Autodesk Fusion 360 part; units mm, degrees
note: some values were not read from the file. Chosen so that the rebuilt part matches the saved one: that a step has no effect.
(part 2 of 3)
sketch "Esquisse23" plane through (0, 78.1168, 0) normal (0, 1, 0) x (-1, 0, 0)
  arc A0 (-120.0939, -5.0643) -> (-115.0939, -10.0643) centre (-115.0939, -5.0643) ccw
  line L0 (-115.0939, -10.0643) -> (-5.0939, -10.0643)
  arc A1 (-5.0939, -10.0643) -> (-0.0939, -5.0643) centre (-5.0939, -5.0643) ccw
  line L1 (-0.0939, -5.0643) -> (-0.0939, 142.9357)
  arc A2 (-0.0939, 142.9357) -> (-5.0939, 147.9357) centre (-5.0939, 142.9357) ccw
  line L2 (-5.0939, 147.9357) -> (-115.0939, 147.9357)
  arc A3 (-115.0939, 147.9357) -> (-120.0939, 142.9357) centre (-115.0939, 142.9357) ccw
  line L3 (-120.0939, 142.9357) -> (-120.0939, -5.0643)
  line L4 (-52.5939, 55.5607) -> (-52.5939, 82.3107)
  line L5 (-52.5939, 82.3107) -> (-37.5939, 82.3107)
  line L6 (-37.5939, 82.3107) -> (-37.5939, 55.5607)
  line L7 (-37.5939, 55.5607) -> (-52.5939, 55.5607)
  circle A4 centre (-17.488, 58.9355) radius 2.625
  circle A5 centre (-17.4939, 78.9357) radius 2.6
  spline S0 degree 3 poles (-59.3641, 46.4248) (-58.9648, 44.9472) (-58.6266, 42.1699) (-58.7596, 41.7802) knots 0 0 0 0 1 1 1 1
  spline S1 degree 3 poles (-58.7596, 41.7802) (-58.8164, 41.6787) (-59.2704, 41.5542) (-59.7808, 41.5574) knots 0 0 0 0 1 1 1 1
  line L8 (-59.7808, 41.5574) -> (-60.6789, 41.5163)
  line L9 (-60.6789, 41.5163) -> (-60.7105, 42.3931)
  spline S2 degree 3 poles (-60.7105, 42.3931) (-60.7436, 43.9055) (-61.4034, 46.4895) (-62.2511, 48.405) knots 0 0 0 0 1 1 1 1
  spline S3 degree 3 poles (-62.2511, 48.405) (-64.5962, 53.7047) (-70.1315, 57.6435) (-75.845, 58.0167) knots 0 0 0 0 1 1 1 1
  spline S4 degree 3 poles (-75.845, 58.0167) (-77.6833, 58.1449) (-77.7447, 58.1686) (-77.7767, 58.8162) knots 0 0 0 0 1 1 1 1
  spline S5 degree 3 poles (-77.7767, 58.8162) (-77.8384, 60.1633) (-77.7414, 60.2317) (-75.8511, 60.101) knots 0 0 0 0 1 1 1 1
  spline S6 degree 3 poles (-75.8511, 60.101) (-74.9059, 60.0357) (-73.7057, 59.8541) (-73.2333, 59.7068) knots 0 0 0 0 1 1 1 1
  spline S7 degree 3 poles (-73.2333, 59.7068) (-72.7396, 59.569) (-71.9177, 59.3219) (-71.4121, 59.2147) knots 0 0 0 0 1 1 1 1
  spline S8 degree 3 poles (-71.4121, 59.2147) (-69.3523, 58.701) (-65.4571, 56.2252) (-63.7728, 54.3745) knots 0 0 0 0 1 1 1 1
  spline S9 degree 3 poles (-63.7728, 54.3745) (-63.367, 53.9177) (-62.7091, 53.0636) (-62.2988, 52.4816) knots 0 0 0 0 1 1 1 1
  spline S10 degree 3 poles (-62.2988, 52.4816) (-61.8886, 51.8996) (-61.4194, 51.2419) (-61.2732, 51.0266) knots 0 0 0 0 1 1 1 1
  spline S11 degree 3 poles (-61.2732, 51.0266) (-60.7168, 50.2293) (-59.7139, 47.848) (-59.3641, 46.4248) knots 0 0 0 0 1 1 1 1
  spline S12 degree 3 poles (-64.0578, 43.2279) (-63.857, 41.7388) (-63.895, 41.5947) (-64.3772, 41.5341) knots 0 0 0 0 1 1 1 1
  spline S13 degree 3 poles (-64.3772, 41.5341) (-65.2896, 41.4103) (-65.4382, 41.5736) (-65.639, 43.0627) knots 0 0 0 0 1 1 1 1
  spline S14 degree 3 poles (-65.639, 43.0627) (-65.9406, 45.0671) (-67.2358, 47.879) (-68.5238, 49.2943) knots 0 0 0 0 1 1 1 1
  spline S15 degree 3 poles (-68.5238, 49.2943) (-70.6445, 51.6136) (-73.2088, 52.9222) (-76.1859, 53.2082) knots 0 0 0 0 1 1 1 1
  spline S16 degree 3 poles (-76.1859, 53.2082) (-77.0153, 53.2993) (-77.698, 53.4044) (-77.7075, 53.4257) knots 0 0 0 0 1 1 1 1
  spline S17 degree 3 poles (-77.7075, 53.4257) (-77.8299, 53.7024) (-77.6934, 54.8318) (-77.5444, 54.8977) knots 0 0 0 0 1 1 1 1
  spline S18 degree 3 poles (-77.5444, 54.8977) (-76.991, 55.1426) (-74.5599, 54.7676) (-72.8996, 54.1789) knots 0 0 0 0 1 1 1 1
  spline S19 degree 3 poles (-72.8996, 54.1789) (-68.0508, 52.4814) (-64.782, 48.4304) (-64.0578, 43.2279) knots 0 0 0 0 1 1 1 1
  spline S20 degree 3 poles (-68.6528, 42.5689) (-68.581, 41.659) (-68.7398, 41.3851) (-69.3305, 41.4546) knots 0 0 0 0 1 1 1 1
  spline S21 degree 3 poles (-69.3305, 41.4546) (-69.6305, 41.5) (-69.7059, 41.6703) (-69.7944, 42.4455) knots 0 0 0 0 1 1 1 1
  spline S22 degree 3 poles (-69.7944, 42.4455) (-69.906, 43.6178) (-70.7724, 45.5759) (-71.5933, 46.5107) knots 0 0 0 0 1 1 1 1
  spline S23 degree 3 poles (-71.5933, 46.5107) (-72.6029, 47.6419) (-74.265, 48.6371) (-75.7296, 48.9562) knots 0 0 0 0 1 1 1 1
  spline S24 degree 3 poles (-75.7296, 48.9562) (-76.4619, 49.1157) (-77.1873, 49.2019) (-77.315, 49.1454) knots 0 0 0 0 1 1 1 1
  spline S25 degree 3 poles (-77.315, 49.1454) (-77.5917, 49.023) (-77.8013, 49.4392) (-77.7249, 49.9566) knots 0 0 0 0 1 1 1 1
  spline S26 degree 3 poles (-77.7249, 49.9566) (-77.677, 50.3087) (-77.5186, 50.3533) (-76.6774, 50.2929) knots 0 0 0 0 1 1 1 1
  spline S27 degree 3 poles (-76.6774, 50.2929) (-75.6283, 50.2226) (-73.453, 49.5055) (-72.5229, 48.899) knots 0 0 0 0 1 1 1 1
  spline S28 degree 3 poles (-72.5229, 48.899) (-70.7429, 47.7523) (-68.8079, 44.5873) (-68.6528, 42.5689) knots 0 0 0 0 1 1 1 1
  spline S29 degree 3 poles (-74.9422, 33.143) (-74.9747, 29.1328) (-75.0002, 25.0493) (-75.0041, 24.0804) knots 0 0 0 0 1 1 1 1
  spline S30 degree 3 poles (-75.0041, 24.0804) (-75.0199, 23.0808) (-75.059, 19.3731) (-75.0694, 15.8307) knots 0 0 0 0 1 1 1 1
  spline S31 degree 3 poles (-75.0694, 15.8307) (-75.1114, 10.2892) (-75.1862, 9.3653) (-75.5906, 9.1864) knots 0 0 0 0 1 1 1 1
  spline S32 degree 3 poles (-75.5906, 9.1864) (-76.2078, 8.9133) (-76.817, 9.2545) (-76.8891, 9.9352) knots 0 0 0 0 1 1 1 1
  spline S33 degree 3 poles (-76.8891, 9.9352) (-76.9383, 10.2189) (-76.9291, 11.521) (-76.9105, 12.8018) knots 0 0 0 0 1 1 1 1
  spline S34 degree 3 poles (-76.9105, 12.8018) (-76.838, 15.2263) (-76.7795, 22.2258) (-76.7274, 31.0805) knots 0 0 0 0 1 1 1 1
  spline S35 degree 3 poles (-76.7274, 31.0805) (-76.7275, 33.9565) (-76.6985, 37.227) (-76.6779, 38.3306) knots 0 0 0 0 1 1 1 1
  spline S36 degree 3 poles (-76.6779, 38.3306) (-76.6109, 41.7452) (-77.5591, 42.8527) (-80.4187, 42.7581) knots 0 0 0 0 1 1 1 1
  spline S37 degree 3 poles (-80.4187, 42.7581) (-81.2955, 42.7264) (-82.6307, 42.6955) (-83.401, 42.7109) knots 0 0 0 0 1 1 1 1
  spline S38 degree 3 poles (-83.401, 42.7109) (-87.5058, 42.727) (-93.9691, 42.6665) (-107.0636, 42.5222) knots 0 0 0 0 1 1 1 1
  spline S39 degree 3 poles (-107.0636, 42.5222) (-109.3583, 42.474) (-110.375, 42.1258) (-110.9864, 41.0918) knots 0 0 0 0 1 1 1 1
  spline S40 degree 3 poles (-110.9864, 41.0918) (-111.4296, 40.3103) (-111.4345, 40.2063) (-111.4267, 33.287) knots 0 0 0 0 1 1 1 1
  spline S41 degree 3 poles (-111.4267, 33.287) (-111.4378, 30.8388) (-111.4136, 28.2534) (-111.436, 27.5563) knots 0 0 0 0 1 1 1 1
  spline S42 degree 3 poles (-111.436, 27.5563) (-111.4418, 25.4413) (-111.443, 15.8965) (-111.4485, 5.1537) knots 0 0 0 0 1 1 1 1
  spline S43 degree 3 poles (-111.4485, 5.1537) (-111.441, -0.4423) (-111.4983, -5.2016) (-111.5388, -5.3977) knots 0 0 0 0 1 1 1 1
  spline S44 degree 3 poles (-111.5388, -5.3977) (-111.698, -5.9008) (-112.3553, -6.1408) (-112.7991, -5.8281) knots 0 0 0 0 1 1 1 1
  spline S45 degree 3 poles (-112.7991, -5.8281) (-113.231, -5.4848) (-113.2035, -6.0071) (-113.2071, 3.4338) knots 0 0 0 0 1 1 1 1
  spline S46 degree 3 poles (-113.2071, 3.4338) (-113.2025, 7.737) (-113.2023, 13.7182) (-113.2069, 16.7194) knots 0 0 0 0 1 1 1 1
  spline S47 degree 3 poles (-113.2069, 16.7194) (-113.1903, 19.73) (-113.1812, 23.9081) (-113.1967, 26.0137) knots 0 0 0 0 1 1 1 1
  spline S48 degree 3 poles (-113.1967, 26.0137) (-113.1815, 28.1074) (-113.1773, 32.1815) (-113.1892, 35.0267) knots 0 0 0 0 1 1 1 1
  spline S49 degree 3 poles (-113.1892, 35.0267) (-113.2201, 40.7905) (-112.989, 41.9363) (-111.5029, 43.1793) knots 0 0 0 0 1 1 1 1
  spline S50 degree 3 poles (-111.5029, 43.1793) (-110.3766, 44.0849) (-109.5445, 44.275) (-106.0115, 44.2858) knots 0 0 0 0 1 1 1 1
  spline S51 degree 3 poles (-106.0115, 44.2858) (-104.3857, 44.2926) (-102.436, 44.3155) (-101.6845, 44.3426) knots 0 0 0 0 1 1 1 1
  spline S52 degree 3 poles (-101.6845, 44.3426) (-100.9236, 44.3485) (-99.2031, 44.3717) (-97.8798, 44.3719) knots 0 0 0 0 1 1 1 1
  spline S53 degree 3 poles (-97.8798, 44.3719) (-96.5564, 44.3722) (-94.784, 44.3929) (-93.9498, 44.4058) knots 0 0 0 0 1 1 1 1
  spline S54 degree 3 poles (-93.9498, 44.4058) (-93.1156, 44.4186) (-91.7497, 44.4377) (-90.8966, 44.4079) knots 0 0 0 0 1 1 1 1
  spline S55 degree 3 poles (-90.8966, 44.4079) (-90.053, 44.3995) (-87.1132, 44.4278) (-84.36, 44.4754) knots 0 0 0 0 1 1 1 1
  spline S56 degree 3 poles (-84.36, 44.4754) (-77.5917, 44.5944) (-76.3092, 44.1693) (-75.3563, 41.6132) knots 0 0 0 0 1 1 1 1
  spline S57 degree 3 poles (-75.3563, 41.6132) (-74.9963, 40.6272) (-74.9232, 39.0816) (-74.9422, 33.143) knots 0 0 0 0 1 1 1 1
  spline S58 degree 3 poles (-107.0966, 36.7302) (-107.157, 35.889) (-107.6232, 35.5046) (-108.0408, 35.9306) knots 0 0 0 0 1 1 1 1
  spline S59 degree 3 poles (-108.0408, 35.9306) (-108.2107, 36.0845) (-108.5865, 36.0709) (-109.0003, 35.9133) knots 0 0 0 0 1 1 1 1
  line L10 (-109.0003, 35.9133) -> (-109.6695, 35.6426)
  line L11 (-109.6695, 35.6426) -> (-109.1251, 36.138)
  spline S60 degree 3 poles (-109.1251, 36.138) (-108.3938, 36.8434) (-108.3861, 37.2285) (-109.0807, 37.3029) knots 0 0 0 0 1 1 1 1
  spline S61 degree 3 poles (-109.0807, 37.3029) (-109.9526, 37.3752) (-109.1983, 37.6836) (-108.0616, 37.703) knots 0 0 0 0 1 1 1 1
  spline S62 degree 3 poles (-108.0616, 37.703) (-107.0194, 37.7061) (-107.0382, 37.7486) (-107.0966, 36.7302) knots 0 0 0 0 1 1 1 1
  spline S63 degree 3 poles (-107.2434, 33.6111) (-107.286, 33.5922) (-107.3564, 33.8665) (-107.3819, 34.2115) knots 0 0 0 0 1 1 1 1
  spline S64 degree 3 poles (-107.3819, 34.2115) (-107.416, 35.0363) (-107.4254, 35.0576) (-107.8085, 34.8881) knots 0 0 0 0 1 1 1 1
  spline S65 degree 3 poles (-107.8085, 34.8881) (-107.9575, 34.8222) (-108.1376, 34.5389) (-108.1711, 34.2695) knots 0 0 0 0 1 1 1 1
  spline S66 degree 3 poles (-108.1711, 34.2695) (-108.2426, 33.8561) (-108.2734, 33.868) (-108.3766, 34.3313) knots 0 0 0 0 1 1 1 1
  spline S67 degree 3 poles (-108.3766, 34.3313) (-108.4327, 34.6882) (-108.6427, 34.8753) (-109.0066, 34.8924) knots 0 0 0 0 1 1 1 1
  spline S68 degree 3 poles (-109.0066, 34.8924) (-109.7958, 34.9504) (-109.545, 35.1886) (-108.5925, 35.2793) knots 0 0 0 0 1 1 1 1
  spline S69 degree 3 poles (-108.5925, 35.2793) (-107.2429, 35.3929) (-107.0399, 35.2791) (-107.1122, 34.4072) knots 0 0 0 0 1 1 1 1
  spline S70 degree 3 poles (-107.1122, 34.4072) (-107.1317, 33.9914) (-107.2009, 33.6299) (-107.2434, 33.6111) knots 0 0 0 0 1 1 1 1
  spline S71 degree 3 poles (-107.1524, 32.8878) (-107.4504, 32.7559) (-109.6338, 32.8587) (-109.565, 32.9909) knots 0 0 0 0 1 1 1 1
  spline S72 degree 3 poles (-109.565, 32.9909) (-109.4701, 33.2366) (-107.2557, 33.3511) (-107.1521, 33.117) knots 0 0 0 0 1 1 1 1
  spline S73 degree 3 poles (-107.1521, 33.117) (-107.105, 33.0106) (-107.1099, 32.9066) (-107.1524, 32.8878) knots 0 0 0 0 1 1 1 1
  spline S74 degree 3 poles (-107.3093, 30.8841) (-107.5462, 30.4993) (-107.8135, 30.3556) (-108.2838, 30.3256) knots 0 0 0 0 1 1 1 1
  spline S75 degree 3 poles (-108.2838, 30.3256) (-109.0566, 30.289) (-109.5426, 30.8121) (-109.5341, 31.6557) knots 0 0 0 0 1 1 1 1
  spline S76 degree 3 poles (-109.5341, 31.6557) (-109.5285, 32.2181) (-109.4409, 32.3078) (-108.9399, 32.3259) knots 0 0 0 0 1 1 1 1
  spline S77 degree 3 poles (-108.9399, 32.3259) (-108.6161, 32.3419) (-108.0725, 32.3788) (-107.7487, 32.3949) knots 0 0 0 0 1 1 1 1
  spline S78 degree 3 poles (-107.7487, 32.3949) (-106.9972, 32.422) (-106.7928, 31.6726) (-107.3093, 30.8841) knots 0 0 0 0 1 1 1 1
  spline S79 degree 3 poles (-107.0664, 27.632) (-107.1494, 27.4171) (-107.3578, 27.1976) (-107.528, 27.1223) knots 0 0 0 0 1 1 1 1
  spline S80 degree 3 poles (-107.528, 27.1223) (-107.8354, 27.0117) (-107.833, 27.0637) (-107.6173, 27.4391) knots 0 0 0 0 1 1 1 1
  spline S81 degree 3 poles (-107.6173, 27.4391) (-107.2523, 28.1097) (-107.6577, 28.7956) (-108.3502, 28.6928) knots 0 0 0 0 1 1 1 1
  spline S82 degree 3 poles (-108.3502, 28.6928) (-109.1492, 28.5428) (-109.3649, 28.1674) (-108.9546, 27.5854) knots 0 0 0 0 1 1 1 1
  spline S83 degree 3 poles (-108.9546, 27.5854) (-108.7495, 27.2944) (-108.7474, 27.1172) (-108.9152, 27.0938) knots 0 0 0 0 1 1 1 1
  spline S84 degree 3 poles (-108.9152, 27.0938) (-109.7425, 27.0077) (-109.7469, 28.6856) (-108.8955, 29.0623) knots 0 0 0 0 1 1 1 1
  spline S85 degree 3 poles (-108.8955, 29.0623) (-108.0016, 29.4579) (-106.746, 28.4609) (-107.0664, 27.632) knots 0 0 0 0 1 1 1 1
  spline S86 degree 3 poles (-107.8998, 25.2017) (-108.3467, 25.0039) (-108.9378, 24.8441) (-109.219, 24.847) knots 0 0 0 0 1 1 1 1
  spline S87 degree 3 poles (-109.219, 24.847) (-109.6987, 24.8383) (-109.7081, 24.8596) (-109.2612, 25.0573) knots 0 0 0 0 1 1 1 1
  spline S88 degree 3 poles (-109.2612, 25.0573) (-108.7172, 25.3235) (-108.7489, 26.2003) (-109.2991, 26.4658) knots 0 0 0 0 1 1 1 1
  spline S89 degree 3 poles (-109.2991, 26.4658) (-110.0523, 26.8452) (-109.3552, 26.8228) (-108.3515, 26.4525) knots 0 0 0 0 1 1 1 1
  spline S90 degree 3 poles (-108.3515, 26.4525) (-107.0194, 25.973) (-106.89, 25.623) (-107.8998, 25.2017) knots 0 0 0 0 1 1 1 1
  spline S91 degree 3 poles (-107.4597, 22.5968) (-107.6631, 22.4813) (-107.9656, 22.4747) (-108.1568, 22.6191) knots 0 0 0 0 1 1 1 1
  spline S92 degree 3 poles (-108.1568, 22.6191) (-108.348, 22.7636) (-108.7545, 22.7619) (-109.0831, 22.6419) knots 0 0 0 0 1 1 1 1
  spline S93 degree 3 poles (-109.0831, 22.6419) (-109.4237, 22.4912) (-109.5583, 22.508) (-109.395, 22.6566) knots 0 0 0 0 1 1 1 1
  spline S94 degree 3 poles (-109.395, 22.6566) (-109.253, 22.7958) (-108.9359, 23.1143) (-108.685, 23.3526) knots 0 0 0 0 1 1 1 1
  line L12 (-108.685, 23.3526) -> (-108.2471, 23.8009)
  line L13 (-108.2471, 23.8009) -> (-108.9675, 23.9911)
  line L14 (-108.9675, 23.9911) -> (-109.6974, 24.2026)
  line L15 (-109.6974, 24.2026) -> (-109.0568, 24.3079)
  spline S95 degree 3 poles (-109.0568, 24.3079) (-108.7093, 24.3853) (-108.1231, 24.4411) (-107.7781, 24.4665) knots 0 0 0 0 1 1 1 1
  spline S96 degree 3 poles (-107.7781, 24.4665) (-107.1825, 24.501) (-107.1424, 24.4679) (-107.1271, 23.6856) knots 0 0 0 0 1 1 1 1
  spline S97 degree 3 poles (-107.1271, 23.6856) (-107.1066, 23.2366) (-107.2657, 22.7335) (-107.4597, 22.5968) knots 0 0 0 0 1 1 1 1
  spline S98 degree 3 poles (-107.1009, 20.9231) (-107.1515, 20.2898) (-108.185, 19.807) (-108.8817, 20.0587) knots 0 0 0 0 1 1 1 1
  spline S99 degree 3 poles (-108.8817, 20.0587) (-109.3824, 20.2698) (-109.7259, 21.1612) (-109.5218, 21.7352) knots 0 0 0 0 1 1 1 1
  spline S100 degree 3 poles (-109.5218, 21.7352) (-109.3794, 22.1036) (-107.3683, 22.1027) (-107.2082, 21.7409) knots 0 0 0 0 1 1 1 1
  spline S101 degree 3 poles (-107.2082, 21.7409) (-107.1329, 21.5706) (-107.098, 21.2043) (-107.1009, 20.9231) knots 0 0 0 0 1 1 1 1
  spline S102 degree 3 poles (-107.3413, 16.9226) (-107.41, 16.7904) (-107.7219, 16.8051) (-108.0195, 16.9025) knots 0 0 0 0 1 1 1 1
  spline S103 degree 3 poles (-108.0195, 16.9025) (-108.3265, 17.0211) (-108.7662, 16.9793) (-109.0453, 16.8049) knots 0 0 0 0 1 1 1 1
  spline S104 degree 3 poles (-109.0453, 16.8049) (-109.3457, 16.621) (-109.5229, 16.6189) (-109.5037, 16.8056) knots 0 0 0 0 1 1 1 1
  spline S105 degree 3 poles (-109.5037, 16.8056) (-109.4751, 16.971) (-109.2881, 17.181) (-109.0753, 17.2752) knots 0 0 0 0 1 1 1 1
  spline S106 degree 3 poles (-109.0753, 17.2752) (-108.8624, 17.3694) (-108.6304, 17.6502) (-108.5662, 17.9077) knots 0 0 0 0 1 1 1 1
  spline S107 degree 3 poles (-108.5662, 17.9077) (-108.4545, 18.288) (-108.504, 18.3424) (-108.9342, 18.2793) knots 0 0 0 0 1 1 1 1
  spline S108 degree 3 poles (-108.9342, 18.2793) (-109.4495, 18.1785) (-109.8106, 18.4768) (-109.4062, 18.6558) knots 0 0 0 0 1 1 1 1
  spline S109 degree 3 poles (-109.4062, 18.6558) (-109.2785, 18.7123) (-108.7042, 18.7374) (-108.1324, 18.7104) knots 0 0 0 0 1 1 1 1
  spline S110 degree 3 poles (-108.1324, 18.7104) (-107.114, 18.6521) (-107.1046, 18.6308) (-107.1507, 17.8723) knots 0 0 0 0 1 1 1 1
  spline S111 degree 3 poles (-107.1507, 17.8723) (-107.1703, 17.4564) (-107.2631, 17.0336) (-107.3413, 16.9226) knots 0 0 0 0 1 1 1 1
  spline S112 degree 3 poles (-107.1866, 14.675) (-107.2459, 14.5215) (-107.3286, 14.5358) (-107.4133, 14.7274) knots 0 0 0 0 1 1 1 1
  spline S113 degree 3 poles (-107.4133, 14.7274) (-107.4887, 14.8976) (-107.4953, 15.2001) (-107.4241, 15.3843) knots 0 0 0 0 1 1 1 1
  spline S114 degree 3 poles (-107.4241, 15.3843) (-107.2936, 15.7221) (-107.6285, 16.1338) (-107.9477, 15.9925) knots 0 0 0 0 1 1 1 1
  spline S115 degree 3 poles (-107.9477, 15.9925) (-108.0329, 15.9548) (-108.1114, 15.6147) (-108.1285, 15.2508) knots 0 0 0 0 1 1 1 1
  spline S116 degree 3 poles (-108.1285, 15.2508) (-108.115, 14.875) (-108.2005, 14.6081) (-108.2926, 14.6437) knots 0 0 0 0 1 1 1 1
  spline S117 degree 3 poles (-108.2926, 14.6437) (-108.3847, 14.6793) (-108.4457, 14.9323) (-108.4216, 15.2229) knots 0 0 0 0 1 1 1 1
  spline S118 degree 3 poles (-108.4216, 15.2229) (-108.3926, 15.6175) (-108.4892, 15.7783) (-108.8081, 15.8663) knots 0 0 0 0 1 1 1 1
  spline S119 degree 3 poles (-108.8081, 15.8663) (-109.1577, 15.9661) (-109.2359, 15.8552) (-109.2296, 15.3235) knots 0 0 0 0 1 1 1 1
  spline S120 degree 3 poles (-109.2296, 15.3235) (-109.2468, 14.9596) (-109.3253, 14.6194) (-109.4317, 14.5723) knots 0 0 0 0 1 1 1 1
  spline S121 degree 3 poles (-109.4317, 14.5723) (-109.5381, 14.5252) (-109.5967, 14.8301) (-109.5653, 15.2767) knots 0 0 0 0 1 1 1 1
  spline S122 degree 3 poles (-109.5653, 15.2767) (-109.5024, 16.1699) (-109.254, 16.3562) (-108.0157, 16.3187) knots 0 0 0 0 1 1 1 1
  spline S123 degree 3 poles (-108.0157, 16.3187) (-107.184, 16.2796) (-107.1344, 16.2252) (-107.1212, 15.6202) knots 0 0 0 0 1 1 1 1
  spline S124 degree 3 poles (-107.1212, 15.6202) (-107.1171, 15.2657) (-107.1367, 14.8498) (-107.1866, 14.675) knots 0 0 0 0 1 1 1 1
  spline S125 degree 3 poles (-108.3622, 12.5004) (-109.4902, 12.0013) (-110.1304, 12.1252) (-109.2292, 12.6767) knots 0 0 0 0 1 1 1 1
  spline S126 degree 3 poles (-109.2292, 12.6767) (-108.8531, 12.9195) (-108.8363, 13.0542) (-109.1827, 13.6644) knots 0 0 0 0 1 1 1 1
  line L16 (-109.1827, 13.6644) -> (-109.5762, 14.3811)
  line L17 (-109.5762, 14.3811) -> (-108.3575, 13.9278)
  spline S127 degree 3 poles (-108.3575, 13.9278) (-107.6821, 13.6667) (-107.1438, 13.3705) (-107.1605, 13.2358) knots 0 0 0 0 1 1 1 1
  spline S128 degree 3 poles (-107.1605, 13.2358) (-107.1867, 13.1224) (-107.7237, 12.783) (-108.3622, 12.5004) knots 0 0 0 0 1 1 1 1
  spline S129 degree 3 poles (-107.1618, 10.9955) (-107.2418, 9.7385) (-108.8635, 9.3772) (-109.3533, 10.4839) knots 0 0 0 0 1 1 1 1
  spline S130 degree 3 poles (-109.3533, 10.4839) (-109.8242, 11.5481) (-109.6347, 11.8101) (-108.3396, 11.8742) knots 0 0 0 0 1 1 1 1
  spline S131 degree 3 poles (-108.3396, 11.8742) (-107.7133, 11.8968) (-107.1722, 11.8817) (-107.1533, 11.8392) knots 0 0 0 0 1 1 1 1
  spline S132 degree 3 poles (-107.1533, 11.8392) (-107.1345, 11.7966) (-107.1422, 11.4114) (-107.1618, 10.9955) knots 0 0 0 0 1 1 1 1
  spline S133 degree 3 poles (-107.2947, 7.7299) (-107.3561, 7.7536) (-107.4147, 8.0585) (-107.4401, 8.4036) knots 0 0 0 0 1 1 1 1
  spline S134 degree 3 poles (-107.4401, 8.4036) (-107.4833, 9.4789) (-108.1214, 9.4256) (-108.1421, 8.322) knots 0 0 0 0 1 1 1 1
  spline S135 degree 3 poles (-108.1421, 8.322) (-108.1498, 7.9369) (-108.2541, 7.7125) (-108.3626, 7.8427) knots 0 0 0 0 1 1 1 1
  spline S136 degree 3 poles (-108.3626, 7.8427) (-108.4711, 7.9728) (-108.5604, 8.2896) (-108.5269, 8.559) knots 0 0 0 0 1 1 1 1
  spline S137 degree 3 poles (-108.5269, 8.559) (-108.4979, 8.9536) (-108.5757, 9.0719) (-108.8569, 9.0747) knots 0 0 0 0 1 1 1 1
  spline S138 degree 3 poles (-108.8569, 9.0747) (-109.0767, 9.0538) (-109.2355, 8.7799) (-109.2669, 8.3333) knots 0 0 0 0 1 1 1 1
  spline S139 degree 3 poles (-109.2669, 8.3333) (-109.3581, 7.504) (-109.6316, 7.892) (-109.5711, 8.7332) knots 0 0 0 0 1 1 1 1
  spline S140 degree 3 poles (-109.5711, 8.7332) (-109.5352, 9.0545) (-109.5111, 9.3451) (-109.5086, 9.3971) knots 0 0 0 0 1 1 1 1
  spline S141 degree 3 poles (-109.5086, 9.3971) (-109.4967, 9.4278) (-108.9626, 9.486) (-108.3056, 9.4968) knots 0 0 0 0 1 1 1 1
  line L18 (-108.3056, 9.4968) -> (-107.1382, 9.5044)
  line L19 (-107.1382, 9.5044) -> (-107.161, 8.578)
  spline S142 degree 3 poles (-107.161, 8.578) (-107.1736, 8.0889) (-107.2333, 7.7061) (-107.2947, 7.7299) knots 0 0 0 0 1 1 1 1
  spline S143 degree 3 poles (-107.1486, 5.962) (-107.3078, 5.4589) (-108.029, 5.1907) (-108.2079, 5.5951) knots 0 0 0 0 1 1 1 1
  spline S144 degree 3 poles (-108.2079, 5.5951) (-108.3209, 5.8505) (-108.4888, 5.8271) (-108.9312, 5.5041) knots 0 0 0 0 1 1 1 1
  spline S145 degree 3 poles (-108.9312, 5.5041) (-109.2979, 5.24) (-109.5414, 5.1577) (-109.6074, 5.3066) knots 0 0 0 0 1 1 1 1
  spline S146 degree 3 poles (-109.6074, 5.3066) (-109.6639, 5.4343) (-109.4769, 5.6444) (-109.2002, 5.7668) knots 0 0 0 0 1 1 1 1
  spline S147 degree 3 poles (-109.2002, 5.7668) (-108.9235, 5.8892) (-108.6395, 6.1676) (-108.5871, 6.3944) knots 0 0 0 0 1 1 1 1
  spline S148 degree 3 poles (-108.5871, 6.3944) (-108.4873, 6.744) (-108.5769, 6.8316) (-109.0235, 6.863) knots 0 0 0 0 1 1 1 1
  spline S149 degree 3 poles (-109.0235, 6.863) (-110.0207, 6.9308) (-109.5168, 7.2301) (-108.3376, 7.2684) knots 0 0 0 0 1 1 1 1
  spline S150 degree 3 poles (-108.3376, 7.2684) (-107.1583, 7.3067) (-106.8918, 6.9919) (-107.1486, 5.962) knots 0 0 0 0 1 1 1 1
  spline S151 degree 3 poles (-107.7762, 37.3457) (-108.0975, 37.3817) (-108.2804, 36.8172) (-108.0732, 36.3489) knots 0 0 0 0 1 1 1 1
  spline S152 degree 3 poles (-108.0732, 36.3489) (-107.9037, 35.9658) (-107.3573, 36.284) (-107.3872, 36.7543) knots 0 0 0 0 1 1 1 1
  spline S153 degree 3 poles (-107.3872, 36.7543) (-107.4147, 37.2766) (-107.4242, 37.2979) (-107.7762, 37.3457) knots 0 0 0 0 1 1 1 1
  spline S154 degree 3 poles (-108.0495, 31.9818) (-109.0209, 31.9337) (-109.3332, 31.7192) (-109.1448, 31.2935) knots 0 0 0 0 1 1 1 1
  spline S155 degree 3 poles (-109.1448, 31.2935) (-108.7586, 30.4209) (-107.5225, 30.5607) (-107.4477, 31.4846) knots 0 0 0 0 1 1 1 1
  spline S156 degree 3 poles (-107.4477, 31.4846) (-107.4163, 31.9311) (-107.5059, 32.0187) (-108.0495, 31.9818) knots 0 0 0 0 1 1 1 1
  spline S157 degree 3 poles (-108.0403, 25.9794) (-108.227, 25.9986) (-108.4067, 25.9445) (-108.4423, 25.8524) knots 0 0 0 0 1 1 1 1
  spline S158 degree 3 poles (-108.4423, 25.8524) (-108.549, 25.5761) (-108.1782, 25.4857) (-107.9273, 25.724) knots 0 0 0 0 1 1 1 1
  spline S159 degree 3 poles (-107.9273, 25.724) (-107.7309, 25.9127) (-107.7497, 25.9553) (-108.0403, 25.9794) knots 0 0 0 0 1 1 1 1
  spline S160 degree 3 poles (-107.7739, 24.112) (-108.0953, 24.148) (-108.2781, 23.5835) (-108.0709, 23.1153) knots 0 0 0 0 1 1 1 1
  spline S161 degree 3 poles (-108.0709, 23.1153) (-107.9297, 22.796) (-107.6648, 22.8878) (-107.475, 23.379) knots 0 0 0 0 1 1 1 1
  spline S162 degree 3 poles (-107.475, 23.379) (-107.297, 23.8395) (-107.3912, 24.0523) (-107.7739, 24.112) knots 0 0 0 0 1 1 1 1
  spline S163 degree 3 poles (-108.1726, 21.6196) (-109.0871, 21.673) (-109.4161, 21.3238) (-109.0058, 20.7418) knots 0 0 0 0 1 1 1 1
  spline S164 degree 3 poles (-109.0058, 20.7418) (-108.6357, 20.193) (-107.7422, 20.3593) (-107.5237, 21.0159) knots 0 0 0 0 1 1 1 1
  spline S165 degree 3 poles (-107.5237, 21.0159) (-107.3527, 21.5497) (-107.3834, 21.5616) (-108.1726, 21.6196) knots 0 0 0 0 1 1 1 1
  spline S166 degree 3 poles (-107.8376, 18.3319) (-108.1782, 18.1812) (-108.1702, 17.243) (-107.8325, 17.1125) knots 0 0 0 0 1 1 1 1
  spline S167 degree 3 poles (-107.8325, 17.1125) (-107.6176, 17.0294) (-107.323, 17.9742) (-107.4643, 18.2935) knots 0 0 0 0 1 1 1 1
  spline S168 degree 3 poles (-107.4643, 18.2935) (-107.502, 18.3786) (-107.6673, 18.4072) (-107.8376, 18.3319) knots 0 0 0 0 1 1 1 1
  spline S169 degree 3 poles (-108.1078, 13.4784) (-108.2944, 13.4976) (-108.4741, 13.4435) (-108.5097, 13.3514) knots 0 0 0 0 1 1 1 1
  spline S170 degree 3 poles (-108.5097, 13.3514) (-108.6165, 13.0751) (-108.2456, 12.9847) (-107.9947, 13.223) knots 0 0 0 0 1 1 1 1
  spline S171 degree 3 poles (-107.9947, 13.223) (-107.7983, 13.4117) (-107.8171, 13.4543) (-108.1078, 13.4784) knots 0 0 0 0 1 1 1 1
  spline S172 degree 3 poles (-108.3285, 11.4464) (-109.4369, 11.3631) (-109.4795, 11.3443) (-109.2158, 10.7484) knots 0 0 0 0 1 1 1 1
  spline S173 degree 3 poles (-109.2158, 10.7484) (-108.9897, 10.2376) (-108.5362, 10.1328) (-107.8125, 10.4531) knots 0 0 0 0 1 1 1 1
  spline S174 degree 3 poles (-107.8125, 10.4531) (-107.5146, 10.5849) (-107.3435, 11.1187) (-107.4942, 11.4593) knots 0 0 0 0 1 1 1 1
  spline S175 degree 3 poles (-107.4942, 11.4593) (-107.5037, 11.4805) (-107.8794, 11.467) (-108.3285, 11.4464) knots 0 0 0 0 1 1 1 1
  spline S176 degree 3 poles (-107.8774, 6.8612) (-108.2818, 6.6822) (-108.2899, 6.0678) (-107.8956, 5.8096) knots 0 0 0 0 1 1 1 1
  spline S177 degree 3 poles (-107.8956, 5.8096) (-107.7045, 5.6651) (-107.5956, 5.7642) (-107.5052, 6.1351) knots 0 0 0 0 1 1 1 1
  spline S178 degree 3 poles (-107.5052, 6.1351) (-107.3694, 6.806) (-107.473, 7.0401) (-107.8774, 6.8612) knots 0 0 0 0 1 1 1 1
  line L20 (-172.7478, 135.2795) -> (-285.7692, 135.2795)
  line L21 (-285.7692, 135.2795) -> (-285.7692, -50.5423)
  line L22 (-285.7692, -50.5423) -> (-172.7478, -50.5423)
  line L23 (-172.7478, -50.5423) -> (-172.7478, 135.2795)
  constraint horizontal L20
  constraint vertical L21
  constraint horizontal L22
  constraint vertical L23
sketch "Esquisse24" plane through (0, 78.1168, 0) normal (0, 1, 0) x (-1, 0, 0)
  arc A0 (-120.0939, -5.0643) -> (-115.0939, -10.0643) centre (-115.0939, -5.0643) ccw
  line L0 (-115.0939, -10.0643) -> (-5.0939, -10.0643)
  arc A1 (-5.0939, -10.0643) -> (-0.0939, -5.0643) centre (-5.0939, -5.0643) ccw
  line L1 (-0.0939, -5.0643) -> (-0.0939, 142.9357)
  arc A2 (-0.0939, 142.9357) -> (-5.0939, 147.9357) centre (-5.0939, 142.9357) ccw
  line L2 (-5.0939, 147.9357) -> (-115.0939, 147.9357)
  arc A3 (-115.0939, 147.9357) -> (-120.0939, 142.9357) centre (-115.0939, 142.9357) ccw
  line L3 (-120.0939, 142.9357) -> (-120.0939, -5.0643)
  line L4 (-52.5939, 55.5607) -> (-52.5939, 82.3107)
  line L5 (-52.5939, 82.3107) -> (-37.5939, 82.3107)
  line L6 (-37.5939, 82.3107) -> (-37.5939, 55.5607)
  line L7 (-37.5939, 55.5607) -> (-52.5939, 55.5607)
  circle A4 centre (-17.488, 58.9355) radius 2.625
  circle A5 centre (-17.4939, 78.9357) radius 2.6
  spline S0 degree 3 poles (-61.7818, 46.0045) (-61.433, 44.7265) (-61.1344, 42.3234) (-61.2487, 41.9858) knots 0 0 0 0 1 1 1 1
  spline S1 degree 3 poles (-61.2487, 41.9858) (-61.2977, 41.8978) (-61.6903, 41.7891) (-62.1321, 41.7907) knots 0 0 0 0 1 1 1 1
  line L8 (-62.1321, 41.7907) -> (-62.9094, 41.7533)
  line L9 (-62.9094, 41.7533) -> (-62.9386, 42.5121)
  spline S2 degree 3 poles (-62.9386, 42.5121) (-62.9704, 43.8211) (-63.547, 46.0563) (-64.2847, 47.7124) knots 0 0 0 0 1 1 1 1
  spline S3 degree 3 poles (-64.2847, 47.7124) (-66.3257, 52.2945) (-71.125, 55.692) (-76.071, 56.0029) knots 0 0 0 0 1 1 1 1
  spline S4 degree 3 poles (-76.071, 56.0029) (-77.6624, 56.11) (-77.7156, 56.1304) (-77.7447, 56.6908) knots 0 0 0 0 1 1 1 1
  spline S5 degree 3 poles (-77.7447, 56.6908) (-77.8009, 57.8566) (-77.7171, 57.916) (-76.0807, 57.8069) knots 0 0 0 0 1 1 1 1
  spline S6 degree 3 poles (-76.0807, 57.8069) (-75.2625, 57.7524) (-74.2233, 57.5978) (-73.8141, 57.4713) knots 0 0 0 0 1 1 1 1
  spline S7 degree 3 poles (-73.8141, 57.4713) (-73.3866, 57.353) (-72.6746, 57.1409) (-72.2368, 57.0492) knots 0 0 0 0 1 1 1 1
  spline S8 degree 3 poles (-72.2368, 57.0492) (-70.4528, 56.6089) (-67.0762, 54.4742) (-65.6144, 52.876) knots 0 0 0 0 1 1 1 1
  spline S9 degree 3 poles (-65.6144, 52.876) (-65.2623, 52.4815) (-64.691, 51.7436) (-64.3347, 51.2407) knots 0 0 0 0 1 1 1 1
  spline S10 degree 3 poles (-64.3347, 51.2407) (-63.9784, 50.7378) (-63.5709, 50.1695) (-63.4439, 49.9835) knots 0 0 0 0 1 1 1 1
  spline S11 degree 3 poles (-63.4439, 49.9835) (-62.9606, 49.2946) (-62.0876, 47.2356) (-61.7818, 46.0045) knots 0 0 0 0 1 1 1 1
  spline S12 degree 3 poles (-65.8375, 43.2276) (-65.6606, 41.9392) (-65.6932, 41.8144) (-66.1104, 41.7608) knots 0 0 0 0 1 1 1 1
  spline S13 degree 3 poles (-66.1104, 41.7608) (-66.8998, 41.6518) (-67.0288, 41.7928) (-67.2058, 43.0813) knots 0 0 0 0 1 1 1 1
  spline S14 degree 3 poles (-67.2058, 43.0813) (-67.4711, 44.8155) (-68.5981, 47.2466) (-69.7159, 48.4688) knots 0 0 0 0 1 1 1 1
  spline S15 degree 3 poles (-69.7159, 48.4688) (-71.5563, 50.4718) (-73.7786, 51.599) (-76.356, 51.8403) knots 0 0 0 0 1 1 1 1
  spline S16 degree 3 poles (-76.356, 51.8403) (-77.074, 51.9174) (-77.6652, 52.0069) (-77.6734, 52.0253) knots 0 0 0 0 1 1 1 1
  spline S17 degree 3 poles (-77.6734, 52.0253) (-77.7799, 52.2645) (-77.6642, 53.2423) (-77.5354, 53.2997) knots 0 0 0 0 1 1 1 1
  spline S18 degree 3 poles (-77.5354, 53.2997) (-77.0569, 53.5128) (-74.9519, 53.1934) (-73.5136, 52.6874) knots 0 0 0 0 1 1 1 1
  spline S19 degree 3 poles (-73.5136, 52.6874) (-69.3132, 51.2284) (-66.4753, 47.729) (-65.8375, 43.2276) knots 0 0 0 0 1 1 1 1
  spline S20 degree 3 poles (-69.8133, 42.6475) (-69.7493, 41.8601) (-69.8861, 41.6227) (-70.3975, 41.6816) knots 0 0 0 0 1 1 1 1
  spline S21 degree 3 poles (-70.3975, 41.6816) (-70.6573, 41.7203) (-70.7229, 41.8675) (-70.8012, 42.5383) knots 0 0 0 0 1 1 1 1
  spline S22 degree 3 poles (-70.8012, 42.5383) (-70.9002, 43.5527) (-71.6543, 45.2457) (-72.3668, 46.053) knots 0 0 0 0 1 1 1 1
  spline S23 degree 3 poles (-72.3668, 46.053) (-73.243, 47.03) (-74.6837, 47.8879) (-75.952, 48.1609) knots 0 0 0 0 1 1 1 1
  spline S24 degree 3 poles (-75.952, 48.1609) (-76.5862, 48.2974) (-77.2142, 48.3705) (-77.3246, 48.3214) knots 0 0 0 0 1 1 1 1
  spline S25 degree 3 poles (-77.3246, 48.3214) (-77.5639, 48.2148) (-77.7462, 48.5746) (-77.6811, 49.0226) knots 0 0 0 0 1 1 1 1
  spline S26 degree 3 poles (-77.6811, 49.0226) (-77.6405, 49.3274) (-77.5035, 49.3664) (-76.7752, 49.3159) knots 0 0 0 0 1 1 1 1
  spline S27 degree 3 poles (-76.7752, 49.3159) (-75.867, 49.2573) (-73.9827, 48.6412) (-73.1764, 48.1182) knots 0 0 0 0 1 1 1 1
  spline S28 degree 3 poles (-73.1764, 48.1182) (-71.6333, 47.1295) (-69.9518, 44.3942) (-69.8133, 42.6475) knots 0 0 0 0 1 1 1 1
  spline S29 degree 3 poles (-75.2371, 34.4757) (-75.2567, 31.0047) (-75.2701, 27.4702) (-75.2715, 26.6316) knots 0 0 0 0 1 1 1 1
  spline S30 degree 3 poles (-75.2715, 26.6316) (-75.283, 25.7664) (-75.309, 22.5571) (-75.3106, 19.4911) knots 0 0 0 0 1 1 1 1
  spline S31 degree 3 poles (-75.3106, 19.4911) (-75.3352, 14.6946) (-75.398, 13.8948) (-75.7476, 13.7391) knots 0 0 0 0 1 1 1 1
  spline S32 degree 3 poles (-75.7476, 13.7391) (-76.2812, 13.5014) (-76.8092, 13.7955) (-76.8731, 14.3845) knots 0 0 0 0 1 1 1 1
  spline S33 degree 3 poles (-76.8731, 14.3845) (-76.9163, 14.6299) (-76.9111, 15.7569) (-76.8977, 16.8655) knots 0 0 0 0 1 1 1 1
  spline S34 degree 3 poles (-76.8977, 16.8655) (-76.8401, 18.9642) (-76.8042, 25.0227) (-76.7778, 32.6868) knots 0 0 0 0 1 1 1 1
  spline S35 degree 3 poles (-76.7778, 32.6868) (-76.784, 35.176) (-76.7659, 38.0069) (-76.7503, 38.9621) knots 0 0 0 0 1 1 1 1
  spline S36 degree 3 poles (-76.7503, 38.9621) (-76.6996, 41.9177) (-77.5226, 42.8743) (-79.9975, 42.7863) knots 0 0 0 0 1 1 1 1
  spline S37 degree 3 poles (-79.9975, 42.7863) (-80.7563, 42.7571) (-81.9119, 42.7275) (-82.5787, 42.7392) knots 0 0 0 0 1 1 1 1
  spline S38 degree 3 poles (-82.5787, 42.7392) (-86.1316, 42.7444) (-91.7257, 42.6784) (-103.0591, 42.5259) knots 0 0 0 0 1 1 1 1
  spline S39 degree 3 poles (-103.0591, 42.5259) (-105.0452, 42.4792) (-105.9244, 42.1758) (-106.4514, 41.2794) knots 0 0 0 0 1 1 1 1
  spline S40 degree 3 poles (-106.4514, 41.2794) (-106.8333, 40.6021) (-106.8374, 40.5121) (-106.816, 34.5232) knots 0 0 0 0 1 1 1 1
  spline S41 degree 3 poles (-106.816, 34.5232) (-106.8204, 32.4042) (-106.794, 30.1665) (-106.8119, 29.5631) knots 0 0 0 0 1 1 1 1
  spline S42 degree 3 poles (-106.8119, 29.5631) (-106.8124, 27.7325) (-106.7933, 19.4711) (-106.7754, 10.1727) knots 0 0 0 0 1 1 1 1
  spline S43 degree 3 poles (-106.7754, 10.1727) (-106.7571, 5.3293) (-106.7966, 1.2098) (-106.8312, 1.04) knots 0 0 0 0 1 1 1 1
  spline S44 degree 3 poles (-106.8312, 1.04) (-106.9679, 0.6042) (-107.5363, 0.3951) (-107.9211, 0.6648) knots 0 0 0 0 1 1 1 1
  spline S45 degree 3 poles (-107.9211, 0.6648) (-108.2957, 0.9611) (-108.2707, 0.509) (-108.2939, 8.6804) knots 0 0 0 0 1 1 1 1
  spline S46 degree 3 poles (-108.2939, 8.6804) (-108.299, 12.4051) (-108.3115, 17.582) (-108.3218, 20.1796) knots 0 0 0 0 1 1 1 1
  spline S47 degree 3 poles (-108.3218, 20.1796) (-108.3138, 22.7854) (-108.3147, 26.4017) (-108.3326, 28.2242) knots 0 0 0 0 1 1 1 1
  spline S48 degree 3 poles (-108.3326, 28.2242) (-108.3239, 30.0364) (-108.3288, 33.5626) (-108.3452, 36.0253) knots 0 0 0 0 1 1 1 1
  spline S49 degree 3 poles (-108.3452, 36.0253) (-108.3841, 41.014) (-108.1865, 42.0062) (-106.9029, 43.0852) knots 0 0 0 0 1 1 1 1
  spline S50 degree 3 poles (-106.9029, 43.0852) (-105.9299, 43.8714) (-105.2101, 44.0377) (-102.1522, 44.0545) knots 0 0 0 0 1 1 1 1
  spline S51 degree 3 poles (-102.1522, 44.0545) (-100.745, 44.0639) (-99.0576, 44.0878) (-98.4072, 44.1129) knots 0 0 0 0 1 1 1 1
  spline S52 degree 3 poles (-98.4072, 44.1129) (-97.7486, 44.1195) (-96.2595, 44.1433) (-95.1141, 44.1463) knots 0 0 0 0 1 1 1 1
  spline S53 degree 3 poles (-95.1141, 44.1463) (-93.9687, 44.1493) (-92.4346, 44.171) (-91.7126, 44.1839) knots 0 0 0 0 1 1 1 1
  spline S54 degree 3 poles (-91.7126, 44.1839) (-90.9906, 44.1967) (-89.8084, 44.2161) (-89.07, 44.1922) knots 0 0 0 0 1 1 1 1
  spline S55 degree 3 poles (-89.07, 44.1922) (-88.3398, 44.1867) (-85.7953, 44.2174) (-83.4125, 44.2644) knots 0 0 0 0 1 1 1 1
  spline S56 degree 3 poles (-83.4125, 44.2644) (-77.5545, 44.3817) (-76.4436, 44.0165) (-75.6134, 41.8061) knots 0 0 0 0 1 1 1 1
  spline S57 degree 3 poles (-75.6134, 41.8061) (-75.2997, 40.9535) (-75.2332, 39.6158) (-75.2371, 34.4757) knots 0 0 0 0 1 1 1 1
  spline S58 degree 3 poles (-103.0754, 37.5126) (-103.126, 36.7844) (-103.5286, 36.4506) (-103.891, 36.8185) knots 0 0 0 0 1 1 1 1
  spline S59 degree 3 poles (-103.891, 36.8185) (-104.0383, 36.9513) (-104.3636, 36.9388) (-104.7214, 36.8015) knots 0 0 0 0 1 1 1 1
  line L10 (-104.7214, 36.8015) -> (-105.3, 36.5658)
  line L11 (-105.3, 36.5658) -> (-104.83, 36.9957)
  spline S60 degree 3 poles (-104.83, 36.9957) (-104.1984, 37.6078) (-104.1926, 37.9412) (-104.794, 38.0041) knots 0 0 0 0 1 1 1 1
  spline S61 degree 3 poles (-104.794, 38.0041) (-105.5488, 38.0648) (-104.8965, 38.3333) (-103.9127, 38.3525) knots 0 0 0 0 1 1 1 1
  spline S62 degree 3 poles (-103.9127, 38.3525) (-103.0107, 38.3574) (-103.0271, 38.3942) (-103.0754, 37.5126) knots 0 0 0 0 1 1 1 1
  spline S63 degree 3 poles (-103.1959, 34.8126) (-103.2327, 34.7962) (-103.2943, 35.0334) (-103.317, 35.332) knots 0 0 0 0 1 1 1 1
  spline S64 degree 3 poles (-103.317, 35.332) (-103.3483, 36.0458) (-103.3565, 36.0642) (-103.6877, 35.9167) knots 0 0 0 0 1 1 1 1
  spline S65 degree 3 poles (-103.6877, 35.9167) (-103.8165, 35.8593) (-103.9718, 35.6137) (-104.0002, 35.3805) knots 0 0 0 0 1 1 1 1
  spline S66 degree 3 poles (-104.0002, 35.3805) (-104.0613, 35.0225) (-104.0879, 35.0327) (-104.1782, 35.4335) knots 0 0 0 0 1 1 1 1
  spline S67 degree 3 poles (-104.1782, 35.4335) (-104.2276, 35.7424) (-104.4097, 35.9038) (-104.7247, 35.9178) knots 0 0 0 0 1 1 1 1
  spline S68 degree 3 poles (-104.7247, 35.9178) (-105.4079, 35.9664) (-105.1913, 36.1731) (-104.3671, 36.2536) knots 0 0 0 0 1 1 1 1
  spline S69 degree 3 poles (-104.3671, 36.2536) (-103.1992, 36.3548) (-103.0233, 36.2567) (-103.084, 35.5019) knots 0 0 0 0 1 1 1 1
  spline S70 degree 3 poles (-103.084, 35.5019) (-103.1001, 35.1419) (-103.1591, 34.8289) (-103.1959, 34.8126) knots 0 0 0 0 1 1 1 1
  spline S71 degree 3 poles (-103.1156, 34.1867) (-103.3733, 34.072) (-105.2633, 34.1563) (-105.204, 34.2709) knots 0 0 0 0 1 1 1 1
  spline S72 degree 3 poles (-105.204, 34.2709) (-105.1224, 34.4837) (-103.206, 34.5875) (-103.1158, 34.3851) knots 0 0 0 0 1 1 1 1
  spline S73 degree 3 poles (-103.1158, 34.3851) (-103.0748, 34.2931) (-103.0788, 34.2031) (-103.1156, 34.1867) knots 0 0 0 0 1 1 1 1
  spline S74 degree 3 poles (-103.2471, 32.4521) (-103.4514, 32.1185) (-103.6824, 31.9936) (-104.0894, 31.9667) knots 0 0 0 0 1 1 1 1
  spline S75 degree 3 poles (-104.0894, 31.9667) (-104.7583, 31.9334) (-105.18, 32.3851) (-105.1745, 33.1153) knots 0 0 0 0 1 1 1 1
  spline S76 degree 3 poles (-105.1745, 33.1153) (-105.1708, 33.6021) (-105.0952, 33.6799) (-104.6615, 33.6966) knots 0 0 0 0 1 1 1 1
  spline S77 degree 3 poles (-104.6615, 33.6966) (-104.3813, 33.7111) (-103.9109, 33.7443) (-103.6307, 33.7588) knots 0 0 0 0 1 1 1 1
  spline S78 degree 3 poles (-103.6307, 33.7588) (-102.9803, 33.7839) (-102.8018, 33.1356) (-103.2471, 32.4521) knots 0 0 0 0 1 1 1 1
  spline S79 degree 3 poles (-103.03, 29.6378) (-103.1015, 29.4516) (-103.2813, 29.2613) (-103.4285, 29.1957) knots 0 0 0 0 1 1 1 1
  spline S80 degree 3 poles (-103.4285, 29.1957) (-103.6943, 29.0993) (-103.6923, 29.1443) (-103.5065, 29.4697) knots 0 0 0 0 1 1 1 1
  spline S81 degree 3 poles (-103.5065, 29.4697) (-103.192, 30.0509) (-103.5443, 30.6437) (-104.1435, 30.5532) knots 0 0 0 0 1 1 1 1
  spline S82 degree 3 poles (-104.1435, 30.5532) (-104.8347, 30.4218) (-105.0206, 30.0964) (-104.6643, 29.5935) knots 0 0 0 0 1 1 1 1
  spline S83 degree 3 poles (-104.6643, 29.5935) (-104.4861, 29.3421) (-104.4839, 29.1887) (-104.6292, 29.1681) knots 0 0 0 0 1 1 1 1
  spline S84 degree 3 poles (-104.6292, 29.1681) (-105.345, 29.0918) (-105.3523, 30.5441) (-104.6162, 30.8719) knots 0 0 0 0 1 1 1 1
  spline S85 degree 3 poles (-104.6162, 30.8719) (-103.8434, 31.2162) (-102.7545, 30.356) (-103.03, 29.6378) knots 0 0 0 0 1 1 1 1
  spline S86 degree 3 poles (-103.7462, 27.5325) (-104.1327, 27.3604) (-104.6439, 27.2209) (-104.8873, 27.2227) knots 0 0 0 0 1 1 1 1
  spline S87 degree 3 poles (-104.8873, 27.2227) (-105.3025, 27.2142) (-105.3107, 27.2326) (-104.9243, 27.4047) knots 0 0 0 0 1 1 1 1
  spline S88 degree 3 poles (-104.9243, 27.4047) (-104.454, 27.6362) (-104.4833, 28.3951) (-104.9601, 28.6238) knots 0 0 0 0 1 1 1 1
  spline S89 degree 3 poles (-104.9601, 28.6238) (-105.6128, 28.9505) (-105.0094, 28.9326) (-104.1398, 28.6142) knots 0 0 0 0 1 1 1 1
  spline S90 degree 3 poles (-104.1398, 28.6142) (-102.9859, 28.202) (-102.8731, 27.8994) (-103.7462, 27.5325) knots 0 0 0 0 1 1 1 1
  spline S91 degree 3 poles (-103.3598, 25.2788) (-103.5356, 25.1784) (-103.7975, 25.1721) (-103.9632, 25.2967) knots 0 0 0 0 1 1 1 1
  spline S92 degree 3 poles (-103.9632, 25.2967) (-104.129, 25.4213) (-104.4808, 25.419) (-104.765, 25.3145) knots 0 0 0 0 1 1 1 1
  spline S93 degree 3 poles (-104.765, 25.3145) (-105.0595, 25.1833) (-105.1761, 25.1975) (-105.035, 25.3265) knots 0 0 0 0 1 1 1 1
  spline S94 degree 3 poles (-105.035, 25.3265) (-104.9124, 25.4473) (-104.6386, 25.7236) (-104.4219, 25.9304) knots 0 0 0 0 1 1 1 1
  line L12 (-104.4219, 25.9304) -> (-104.0439, 26.3193)
  line L13 (-104.0439, 26.3193) -> (-104.6678, 26.4825)
  line L14 (-104.6678, 26.4825) -> (-105.3, 26.664)
  line L15 (-105.3, 26.664) -> (-104.7458, 26.7565)
  spline S95 degree 3 poles (-104.7458, 26.7565) (-104.4452, 26.8242) (-103.9379, 26.8737) (-103.6393, 26.8965) knots 0 0 0 0 1 1 1 1
  spline S96 degree 3 poles (-103.6393, 26.8965) (-103.1239, 26.9276) (-103.0891, 26.899) (-103.0743, 26.222) knots 0 0 0 0 1 1 1 1
  spline S97 degree 3 poles (-103.0743, 26.222) (-103.0555, 25.8334) (-103.1922, 25.3976) (-103.3598, 25.2788) knots 0 0 0 0 1 1 1 1
  spline S98 degree 3 poles (-103.0457, 23.8309) (-103.0882, 23.2827) (-103.9817, 22.8627) (-104.5852, 23.079) knots 0 0 0 0 1 1 1 1
  spline S99 degree 3 poles (-104.5852, 23.079) (-105.019, 23.2607) (-105.3183, 24.0315) (-105.1428, 24.5287) knots 0 0 0 0 1 1 1 1
  spline S100 degree 3 poles (-105.1428, 24.5287) (-105.0203, 24.8479) (-103.2797, 24.8514) (-103.1404, 24.5386) knots 0 0 0 0 1 1 1 1
  spline S101 degree 3 poles (-103.1404, 24.5386) (-103.0748, 24.3913) (-103.0438, 24.0743) (-103.0457, 23.8309) knots 0 0 0 0 1 1 1 1
  spline S102 degree 3 poles (-103.2453, 20.3679) (-103.3045, 20.2533) (-103.5745, 20.2654) (-103.8323, 20.349) knots 0 0 0 0 1 1 1 1
  spline S103 degree 3 poles (-103.8323, 20.349) (-104.0983, 20.4511) (-104.4787, 20.4139) (-104.7199, 20.2624) knots 0 0 0 0 1 1 1 1
  spline S104 degree 3 poles (-104.7199, 20.2624) (-104.9796, 20.1026) (-105.133, 20.1004) (-105.1168, 20.262) knots 0 0 0 0 1 1 1 1
  spline S105 degree 3 poles (-105.1168, 20.262) (-105.0923, 20.4052) (-104.9309, 20.5874) (-104.7469, 20.6694) knots 0 0 0 0 1 1 1 1
  spline S106 degree 3 poles (-104.7469, 20.6694) (-104.5629, 20.7513) (-104.3626, 20.9949) (-104.3076, 21.2179) knots 0 0 0 0 1 1 1 1
  spline S107 degree 3 poles (-104.3076, 21.2179) (-104.2117, 21.5473) (-104.2547, 21.5943) (-104.6269, 21.5388) knots 0 0 0 0 1 1 1 1
  spline S108 degree 3 poles (-104.6269, 21.5388) (-105.0727, 21.4504) (-105.3859, 21.7079) (-105.0363, 21.8636) knots 0 0 0 0 1 1 1 1
  spline S109 degree 3 poles (-105.0363, 21.8636) (-104.9259, 21.9128) (-104.4288, 21.9357) (-103.9338, 21.9137) knots 0 0 0 0 1 1 1 1
  spline S110 degree 3 poles (-103.9338, 21.9137) (-103.0522, 21.8653) (-103.044, 21.8469) (-103.0824, 21.1903) knots 0 0 0 0 1 1 1 1
  spline S111 degree 3 poles (-103.0824, 21.1903) (-103.0984, 20.8303) (-103.1779, 20.4641) (-103.2453, 20.3679) knots 0 0 0 0 1 1 1 1
  spline S112 degree 3 poles (-103.1066, 18.4228) (-103.1577, 18.2898) (-103.2293, 18.3021) (-103.303, 18.4677) knots 0 0 0 0 1 1 1 1
  spline S113 degree 3 poles (-103.303, 18.4677) (-103.3686, 18.6149) (-103.375, 18.8767) (-103.3137, 19.0363) knots 0 0 0 0 1 1 1 1
  spline S114 degree 3 poles (-103.3137, 19.0363) (-103.2015, 19.3289) (-103.4922, 19.6845) (-103.7683, 19.5616) knots 0 0 0 0 1 1 1 1
  spline S115 degree 3 poles (-103.7683, 19.5616) (-103.8419, 19.5288) (-103.9091, 19.2342) (-103.9232, 18.9192) knots 0 0 0 0 1 1 1 1
  spline S116 degree 3 poles (-103.9232, 18.9192) (-103.9106, 18.594) (-103.9841, 18.3628) (-104.0639, 18.3934) knots 0 0 0 0 1 1 1 1
  spline S117 degree 3 poles (-104.0639, 18.3934) (-104.1437, 18.424) (-104.197, 18.6428) (-104.1768, 18.8944) knots 0 0 0 0 1 1 1 1
  spline S118 degree 3 poles (-104.1768, 18.8944) (-104.1525, 19.236) (-104.2365, 19.3751) (-104.5127, 19.4505) knots 0 0 0 0 1 1 1 1
  spline S119 degree 3 poles (-104.5127, 19.4505) (-104.8155, 19.5362) (-104.8829, 19.44) (-104.8764, 18.9798) knots 0 0 0 0 1 1 1 1
  spline S120 degree 3 poles (-104.8764, 18.9798) (-104.8904, 18.6648) (-104.9577, 18.3702) (-105.0497, 18.3292) knots 0 0 0 0 1 1 1 1
  spline S121 degree 3 poles (-105.0497, 18.3292) (-105.1417, 18.2882) (-105.1931, 18.552) (-105.1668, 18.9386) knots 0 0 0 0 1 1 1 1
  spline S122 degree 3 poles (-105.1668, 18.9386) (-105.1143, 19.7118) (-104.8996, 19.8736) (-103.8278, 19.8438) knots 0 0 0 0 1 1 1 1
  spline S123 degree 3 poles (-103.8278, 19.8438) (-103.1078, 19.8117) (-103.0648, 19.7647) (-103.0521, 19.241) knots 0 0 0 0 1 1 1 1
  spline S124 degree 3 poles (-103.0521, 19.241) (-103.0478, 18.9342) (-103.0638, 18.5742) (-103.1066, 18.4228) knots 0 0 0 0 1 1 1 1
  spline S125 degree 3 poles (-104.1196, 16.5382) (-105.0949, 16.1038) (-105.6493, 16.2097) (-104.8704, 16.6889) knots 0 0 0 0 1 1 1 1
  spline S126 degree 3 poles (-104.8704, 16.6889) (-104.5453, 16.8999) (-104.5311, 17.0165) (-104.8322, 17.5439) knots 0 0 0 0 1 1 1 1
  line L16 (-104.8322, 17.5439) -> (-105.1743, 18.1634)
  line L17 (-105.1743, 18.1634) -> (-104.1186, 17.7736)
  spline S127 degree 3 poles (-104.1186, 17.7736) (-103.5334, 17.5491) (-103.0668, 17.2938) (-103.0811, 17.1772) knots 0 0 0 0 1 1 1 1
  spline S128 degree 3 poles (-103.0811, 17.1772) (-103.1035, 17.079) (-103.5675, 16.7841) (-104.1196, 16.5382) knots 0 0 0 0 1 1 1 1
  spline S129 degree 3 poles (-103.0774, 15.2382) (-103.144, 14.15) (-104.5469, 13.8338) (-104.9731, 14.7907) knots 0 0 0 0 1 1 1 1
  spline S130 degree 3 poles (-104.9731, 14.7907) (-105.383, 15.7108) (-105.2195, 15.938) (-104.0987, 15.9962) knots 0 0 0 0 1 1 1 1
  spline S131 degree 3 poles (-104.0987, 15.9962) (-103.5567, 16.0171) (-103.0883, 16.0052) (-103.0719, 15.9684) knots 0 0 0 0 1 1 1 1
  spline S132 degree 3 poles (-103.0719, 15.9684) (-103.0555, 15.9316) (-103.0614, 15.5982) (-103.0774, 15.2382) knots 0 0 0 0 1 1 1 1
  spline S133 degree 3 poles (-103.1855, 12.4113) (-103.2387, 12.4318) (-103.2901, 12.6956) (-103.3128, 12.9942) knots 0 0 0 0 1 1 1 1
  spline S134 degree 3 poles (-103.3128, 12.9942) (-103.3525, 13.9248) (-103.9047, 13.8773) (-103.9202, 12.9221) knots 0 0 0 0 1 1 1 1
  spline S135 degree 3 poles (-103.9202, 12.9221) (-103.9261, 12.5887) (-104.0159, 12.3943) (-104.1101, 12.5067) knots 0 0 0 0 1 1 1 1
  spline S136 degree 3 poles (-104.1101, 12.5067) (-104.2043, 12.6191) (-104.2823, 12.8932) (-104.2538, 13.1264) knots 0 0 0 0 1 1 1 1
  spline S137 degree 3 poles (-104.2538, 13.1264) (-104.2296, 13.468) (-104.2971, 13.5702) (-104.5405, 13.572) knots 0 0 0 0 1 1 1 1
  spline S138 degree 3 poles (-104.5405, 13.572) (-104.7307, 13.5534) (-104.8676, 13.3161) (-104.8939, 12.9295) knots 0 0 0 0 1 1 1 1
  spline S139 degree 3 poles (-104.8939, 12.9295) (-104.971, 12.2115) (-105.2085, 12.5467) (-105.158, 13.2749) knots 0 0 0 0 1 1 1 1
  spline S140 degree 3 poles (-105.158, 13.2749) (-105.1276, 13.5531) (-105.1073, 13.8047) (-105.1053, 13.8497) knots 0 0 0 0 1 1 1 1
  spline S141 degree 3 poles (-105.1053, 13.8497) (-105.0951, 13.8763) (-104.6329, 13.9278) (-104.0643, 13.9385) knots 0 0 0 0 1 1 1 1
  line L18 (-104.0643, 13.9385) -> (-103.0538, 13.9476)
  line L19 (-103.0538, 13.9476) -> (-103.0716, 13.1457)
  spline S142 degree 3 poles (-103.0716, 13.1457) (-103.0815, 12.7223) (-103.1323, 12.3909) (-103.1855, 12.4113) knots 0 0 0 0 1 1 1 1
  spline S143 degree 3 poles (-103.0554, 10.8815) (-103.1921, 10.4457) (-103.8157, 10.212) (-103.9715, 10.5617) knots 0 0 0 0 1 1 1 1
  spline S144 degree 3 poles (-103.9715, 10.5617) (-104.0698, 10.7825) (-104.215, 10.7619) (-104.5973, 10.4814) knots 0 0 0 0 1 1 1 1
  spline S145 degree 3 poles (-104.5973, 10.4814) (-104.9141, 10.252) (-105.1248, 10.1803) (-105.1821, 10.3091) knots 0 0 0 0 1 1 1 1
  spline S146 degree 3 poles (-105.1821, 10.3091) (-105.2313, 10.4195) (-105.0699, 10.6017) (-104.8307, 10.7082) knots 0 0 0 0 1 1 1 1
  spline S147 degree 3 poles (-104.8307, 10.7082) (-104.5914, 10.8148) (-104.3462, 11.0563) (-104.3013, 11.2527) knots 0 0 0 0 1 1 1 1
  spline S148 degree 3 poles (-104.3013, 11.2527) (-104.2157, 11.5555) (-104.2935, 11.6311) (-104.6801, 11.6574) knots 0 0 0 0 1 1 1 1
  spline S149 degree 3 poles (-104.6801, 11.6574) (-105.5433, 11.714) (-105.1078, 11.9741) (-104.0872, 12.0097) knots 0 0 0 0 1 1 1 1
  spline S150 degree 3 poles (-104.0872, 12.0097) (-103.0666, 12.0453) (-102.8352, 11.7735) (-103.0554, 10.8815) knots 0 0 0 0 1 1 1 1
  spline S151 degree 3 poles (-103.6649, 38.0439) (-103.9431, 38.0743) (-104.1002, 37.5854) (-103.9199, 37.1805) knots 0 0 0 0 1 1 1 1
  spline S152 degree 3 poles (-103.9199, 37.1805) (-103.7724, 36.8493) (-103.3001, 37.1258) (-103.327, 37.5328) knots 0 0 0 0 1 1 1 1
  spline S153 degree 3 poles (-103.327, 37.5328) (-103.352, 37.9848) (-103.3601, 38.0032) (-103.6649, 38.0439) knots 0 0 0 0 1 1 1 1
  spline S154 degree 3 poles (-103.8902, 33.4006) (-104.7308, 33.357) (-105.0006, 33.1706) (-104.8367, 32.8026) knots 0 0 0 0 1 1 1 1
  spline S155 degree 3 poles (-104.8367, 32.8026) (-104.5006, 32.0481) (-103.431, 32.1717) (-103.3682, 32.9715) knots 0 0 0 0 1 1 1 1
  spline S156 degree 3 poles (-103.3682, 32.9715) (-103.342, 33.3582) (-103.4198, 33.4338) (-103.8902, 33.4006) knots 0 0 0 0 1 1 1 1
  spline S157 degree 3 poles (-103.8695, 28.2054) (-104.0311, 28.2216) (-104.1865, 28.1744) (-104.2171, 28.0946) knots 0 0 0 0 1 1 1 1
  spline S158 degree 3 poles (-104.2171, 28.0946) (-104.309, 27.8552) (-103.9878, 27.7778) (-103.7711, 27.9845) knots 0 0 0 0 1 1 1 1
  spline S159 degree 3 poles (-103.7711, 27.9845) (-103.6015, 28.1483) (-103.6179, 28.1851) (-103.8695, 28.2054) knots 0 0 0 0 1 1 1 1
  spline S160 degree 3 poles (-103.635, 26.5897) (-103.9132, 26.6201) (-104.0703, 26.1312) (-103.89, 25.7263) knots 0 0 0 0 1 1 1 1
  spline S161 degree 3 poles (-103.89, 25.7263) (-103.767, 25.4503) (-103.538, 25.5302) (-103.3747, 25.9558) knots 0 0 0 0 1 1 1 1
  spline S162 degree 3 poles (-103.3747, 25.9558) (-103.2216, 26.3548) (-103.3036, 26.5388) (-103.635, 26.5897) knots 0 0 0 0 1 1 1 1
  spline S163 degree 3 poles (-103.9748, 24.4315) (-104.7664, 24.4758) (-105.0505, 24.1729) (-104.6941, 23.67) knots 0 0 0 0 1 1 1 1
  spline S164 degree 3 poles (-104.6941, 23.67) (-104.3726, 23.1958) (-103.5996, 23.3416) (-103.4119, 23.9104) knots 0 0 0 0 1 1 1 1
  spline S165 degree 3 poles (-103.4119, 23.9104) (-103.265, 24.3728) (-103.2916, 24.383) (-103.9748, 24.4315) knots 0 0 0 0 1 1 1 1
  spline S166 degree 3 poles (-103.6779, 21.5866) (-103.9723, 21.4554) (-103.9635, 20.6434) (-103.6709, 20.5312) knots 0 0 0 0 1 1 1 1
  spline S167 degree 3 poles (-103.6709, 20.5312) (-103.4847, 20.4597) (-103.2317, 21.2781) (-103.3547, 21.5541) knots 0 0 0 0 1 1 1 1
  spline S168 degree 3 poles (-103.3547, 21.5541) (-103.3875, 21.6277) (-103.5307, 21.6522) (-103.6779, 21.5866) knots 0 0 0 0 1 1 1 1
  spline S169 degree 3 poles (-103.9014, 17.3852) (-104.063, 17.4014) (-104.2185, 17.3542) (-104.2491, 17.2744) knots 0 0 0 0 1 1 1 1